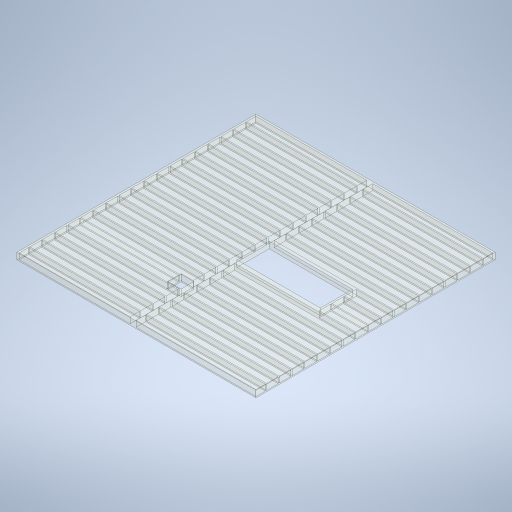
# Autodesk Inventor part: Existing_Basement_And_First_Floor_Transition
Saved by Autodesk Inventor 2024 (Build 280153000, 153)
## iProperties
Created: 2023-05-18
Part Number: Existing_Basement_And_First_Floor_Transition
Material: Wood (Southern Pine)
Document SubType Name: Modeling
Designer: Tom
Density: 7.85 g/cm^3
Appearance: Clear
Mass: 1.71886e+07 g
Surface Area: 1.80544e+06 cm^2
Volume: 2.18963e+06 cm^3
Author: Tom
Autodesk Inventor part; units mm, degrees
ref_plane "YZ Plane" through (0, 0, 0) normal (1, 0, 0) x (0, 1, 0)
ref_plane "XZ Plane" through (0, 0, 0) normal (0, 1, 0) x (-1, 0, 0)
ref_plane "XY Plane" through (0, 0, 0) normal (0, 0, 1) x (1, 0, 0)
sketch "Sketch1" plane through (0, 0, 0) normal (0, 1, 0) x (-1, 0, 0)
  line L0 (0, 0) -> (7620, 0)
  line L1 (7620, 0) -> (7620, -7620)
  line L2 (7620, -7620) -> (0, -7620)
  line L3 (0, -7620) -> (0, 0)
  line L4 (7581.9, -7581.9) -> (7581.9, -38.1)
  line L5 (7581.9, -38.1) -> (38.1, -38.1)
  line L6 (38.1, -38.1) -> (38.1, -7581.9)
  line L7 (38.1, -7581.9) -> (7581.9, -7581.9)
  line L8 (4051.3, -7581.9) -> (4051.3, -38.1)
  line L9 (3860.8, -38.1) -> (3860.8, -7581.9)
  line L10 (7581.9, -336.55) -> (38.1, -336.55)
  line L11 (38.1, -336.55) -> (38.1, -374.65)
  line L12 (38.1, -374.65) -> (7581.9, -374.65)
  line L13 (7581.9, -374.65) -> (7581.9, -336.55)
  line L14 (7581.9, -742.95) -> (38.1, -742.95)
  line L15 (38.1, -781.05) -> (7581.9, -781.05)
  line L16 (7581.9, -781.05) -> (7581.9, -742.95)
  line L17 (38.1, -742.95) -> (38.1, -781.05)
  line L18 (7581.9, -1149.35) -> (38.1, -1149.35)
  line L19 (38.1, -1187.45) -> (7581.9, -1187.45)
  line L20 (7581.9, -1187.45) -> (7581.9, -1149.35)
  line L21 (38.1, -1149.35) -> (38.1, -1187.45)
  line L22 (7581.9, -1555.75) -> (38.1, -1555.75)
  line L23 (38.1, -1593.85) -> (7581.9, -1593.85)
  line L24 (7581.9, -1593.85) -> (7581.9, -1555.75)
  line L25 (38.1, -1555.75) -> (38.1, -1593.85)
  line L26 (7581.9, -1962.15) -> (38.1, -1962.15)
  line L27 (38.1, -2000.25) -> (7581.9, -2000.25)
  line L28 (7581.9, -2000.25) -> (7581.9, -1962.15)
  line L29 (38.1, -1962.15) -> (38.1, -2000.25)
  line L30 (7581.9, -2368.55) -> (38.1, -2368.55)
  line L31 (38.1, -2406.65) -> (7581.9, -2406.65)
  line L32 (7581.9, -2406.65) -> (7581.9, -2368.55)
  line L33 (38.1, -2368.55) -> (38.1, -2406.65)
  line L34 (7581.9, -2774.95) -> (38.1, -2774.95)
  line L35 (38.1, -2813.05) -> (7581.9, -2813.05)
  line L36 (7581.9, -2813.05) -> (7581.9, -2774.95)
  line L37 (38.1, -2774.95) -> (38.1, -2813.05)
  line L38 (7581.9, -3181.35) -> (38.1, -3181.35)
  line L39 (38.1, -3219.45) -> (7581.9, -3219.45)
  line L40 (7581.9, -3219.45) -> (7581.9, -3181.35)
  line L41 (38.1, -3181.35) -> (38.1, -3219.45)
  line L42 (7581.9, -3587.75) -> (38.1, -3587.75)
  line L43 (38.1, -3625.85) -> (7581.9, -3625.85)
  line L44 (7581.9, -3625.85) -> (7581.9, -3587.75)
  line L45 (38.1, -3587.75) -> (38.1, -3625.85)
  line L46 (7581.9, -3994.15) -> (38.1, -3994.15)
  line L47 (38.1, -4032.25) -> (7581.9, -4032.25)
  line L48 (7581.9, -4032.25) -> (7581.9, -3994.15)
  line L49 (38.1, -3994.15) -> (38.1, -4032.25)
  line L50 (7581.9, -4400.55) -> (38.1, -4400.55)
  line L51 (38.1, -4438.65) -> (7581.9, -4438.65)
  line L52 (7581.9, -4438.65) -> (7581.9, -4400.55)
  line L53 (38.1, -4400.55) -> (38.1, -4438.65)
  line L54 (7581.9, -4806.95) -> (38.1, -4806.95)
  line L55 (38.1, -4845.05) -> (7581.9, -4845.05)
  line L56 (7581.9, -4845.05) -> (7581.9, -4806.95)
  line L57 (38.1, -4806.95) -> (38.1, -4845.05)
  line L58 (7581.9, -5213.35) -> (38.1, -5213.35)
  line L59 (38.1, -5251.45) -> (7581.9, -5251.45)
  line L60 (7581.9, -5251.45) -> (7581.9, -5213.35)
  line L61 (38.1, -5213.35) -> (38.1, -5251.45)
  line L62 (7581.9, -5619.75) -> (38.1, -5619.75)
  line L63 (38.1, -5657.85) -> (7581.9, -5657.85)
  line L64 (7581.9, -5657.85) -> (7581.9, -5619.75)
  line L65 (38.1, -5619.75) -> (38.1, -5657.85)
  line L66 (7581.9, -6026.15) -> (38.1, -6026.15)
  line L67 (38.1, -6064.25) -> (7581.9, -6064.25)
  line L68 (7581.9, -6064.25) -> (7581.9, -6026.15)
  line L69 (38.1, -6026.15) -> (38.1, -6064.25)
  line L70 (7581.9, -6432.55) -> (38.1, -6432.55)
  line L71 (38.1, -6470.65) -> (7581.9, -6470.65)
  line L72 (7581.9, -6470.65) -> (7581.9, -6432.55)
  line L73 (38.1, -6432.55) -> (38.1, -6470.65)
  line L74 (7581.9, -6838.95) -> (38.1, -6838.95)
  line L75 (38.1, -6877.05) -> (7581.9, -6877.05)
  line L76 (7581.9, -6877.05) -> (7581.9, -6838.95)
  line L77 (38.1, -6838.95) -> (38.1, -6877.05)
  line L78 (7581.9, -7245.35) -> (38.1, -7245.35)
  line L79 (38.1, -7283.45) -> (7581.9, -7283.45)
  line L80 (7581.9, -7283.45) -> (7581.9, -7245.35)
  line L81 (38.1, -7245.35) -> (38.1, -7283.45)
  point P0 (38.1, -7245.35)
  point P1 (38.1, -6838.95)
  point P2 (38.1, -6432.55)
  point P3 (38.1, -6026.15)
  point P4 (38.1, -5619.75)
  point P5 (38.1, -5213.35)
  point P6 (38.1, -4806.95)
  point P7 (38.1, -4400.55)
  point P8 (38.1, -3994.15)
  point P9 (38.1, -3587.75)
  point P10 (38.1, -3181.35)
  point P11 (38.1, -2774.95)
  point P12 (38.1, -2368.55)
  point P13 (38.1, -1962.15)
  point P14 (38.1, -1555.75)
  point P15 (38.1, -1149.35)
  point P16 (38.1, -742.95)
  point P17 (38.1, -336.55)
  point P18 (4051.3, -7283.45)
  point P19 (3860.8, -7283.45)
  point P20 (3860.8, -7245.35)
  point P21 (4051.3, -7245.35)
  point P22 (4051.3, -6877.05)
  point P23 (3860.8, -6877.05)
  point P24 (3860.8, -6838.95)
  point P25 (4051.3, -6838.95)
  point P26 (4051.3, -6470.65)
  point P27 (3860.8, -6470.65)
  point P28 (3860.8, -6432.55)
  point P29 (4051.3, -6432.55)
  point P30 (4051.3, -6064.25)
  point P31 (3860.8, -6064.25)
  point P32 (3860.8, -6026.15)
  point P33 (4051.3, -6026.15)
  point P34 (4051.3, -5657.85)
  point P35 (3860.8, -5657.85)
  point P36 (3860.8, -5619.75)
  point P37 (4051.3, -5619.75)
  point P38 (4051.3, -5251.45)
  point P39 (3860.8, -5251.45)
  point P40 (3860.8, -5213.35)
  point P41 (4051.3, -5213.35)
  point P42 (4051.3, -4845.05)
  point P43 (3860.8, -4845.05)
  point P44 (3860.8, -4806.95)
  point P45 (4051.3, -4806.95)
  point P46 (4051.3, -4438.65)
  point P47 (3860.8, -4438.65)
  point P48 (3860.8, -4400.55)
  point P49 (4051.3, -4400.55)
  point P50 (4051.3, -4032.25)
  point P51 (3860.8, -4032.25)
  point P52 (3860.8, -3994.15)
  point P53 (4051.3, -3994.15)
  point P54 (4051.3, -3625.85)
  point P55 (3860.8, -3625.85)
  point P56 (3860.8, -3587.75)
  point P57 (4051.3, -3587.75)
  point P58 (4051.3, -3219.45)
  point P59 (3860.8, -3219.45)
  point P60 (3860.8, -3181.35)
  point P61 (4051.3, -3181.35)
  point P62 (4051.3, -2813.05)
  point P63 (3860.8, -2813.05)
  point P64 (3860.8, -2774.95)
  point P65 (4051.3, -2774.95)
  point P66 (4051.3, -2406.65)
  point P67 (3860.8, -2406.65)
  point P68 (3860.8, -2368.55)
  point P69 (4051.3, -2368.55)
  point P70 (4051.3, -2000.25)
  point P71 (3860.8, -2000.25)
  point P72 (3860.8, -1962.15)
  point P73 (4051.3, -1962.15)
  point P74 (4051.3, -1593.85)
  point P75 (3860.8, -1593.85)
  point P76 (3860.8, -1555.75)
  point P77 (4051.3, -1555.75)
  point P78 (4051.3, -1187.45)
  point P79 (3860.8, -1187.45)
  point P80 (3860.8, -1149.35)
  point P81 (4051.3, -1149.35)
  point P82 (4051.3, -781.05)
  point P83 (3860.8, -781.05)
  point P84 (3860.8, -742.95)
  point P85 (4051.3, -742.95)
  point P86 (4051.3, -374.65)
  point P87 (3860.8, -374.65)
  point P88 (3860.8, -336.55)
  point P89 (4051.3, -336.55)
  dimension "d10" = 190.5
  dimension "d1" = 7620
  dimension "d3" = 7620
  dimension "d9" = 38.1
  dimension "d11" = 3568.7
  dimension "d12" = 38.1
  dimension "d13" = 336.55
  dimension "d16" = 406.4
  dimension "d21" = 336.55
  constraints: 156 end point, 68 vertical alignment, 39 parallel, 34 collinear, 5 horizontal, 4 point on line, 2 perpendicular, 17 other
  measures "d1" distance of L0.start L0.end
  measures "d3" distance of L2.end L0.start
  measures "d12" distance between parallel lines of L10 L12
  measures "d13" distance between parallel lines of L0 L10
  measures "d16" distance of L10.start L14.start
  measures "d21" distance between parallel lines of L2 L79
extrude "Extrusion1" add sketch "Sketch1" along normal blind 190.5 contours L0 L1 L2 L3 | L79 L8 L78 L4 | L7 L9 L79 L8 | L79 L9 L78 L8 | L75 L8 L74 L4 | L78 L9 L75 L8 | L79 L6 L78 L9 | L75 L9 L74 L8 | L71 L8 L70 L4 | L74 L9 L71 L8 | L75 L6 L74 L9 | L71 L9 L70 L8 | L67 L8 L66 L4 | L70 L9 L67 L8 | L71 L6 L70 L9 | L67 L9 L66 L8 | L63 L8 L62 L4 | L66 L9 L63 L8 | L67 L6 L66 L9 | L63 L9 L62 L8 | L59 L8 L58 L4 | L62 L9 L59 L8 | L63 L6 L62 L9 | L59 L9 L58 L8 | L55 L8 L54 L4 | L58 L9 L55 L8 | L59 L6 L58 L9 | L55 L9 L54 L8 | L51 L8 L50 L4 | L54 L9 L51 L8 | L55 L6 L54 L9 | L51 L9 L50 L8 | L47 L8 L46 L4 | L50 L9 L47 L8 | L51 L6 L50 L9 | L47 L9 L46 L8 | L43 L8 L42 L4 | L46 L9 L43 L8 | L47 L6 L46 L9 | L43 L9 L42 L8 | L39 L8 L38 L4 | L42 L9 L39 L8 | L43 L6 L42 L9 | L39 L9 L38 L8 | L35 L8 L34 L4 | L38 L9 L35 L8 | L39 L6 L38 L9 | L35 L9 L34 L8 | L31 L8 L30 L4 | L34 L9 L31 L8 | L35 L6 L34 L9 | L31 L9 L30 L8 | L27 L8 L26 L4 | L30 L9 L27 L8 | L31 L6 L30 L9 | L27 L9 L26 L8 | L23 L8 L22 L4 | L26 L9 L23 L8 | L27 L6 L26 L9 | L23 L9 L22 L8 | L19 L8 L18 L4 | L22 L9 L19 L8 | L23 L6 L22 L9 | L19 L9 L18 L8 | L15 L8 L14 L4 | L18 L9 L15 L8 | L19 L6 L18 L9 | L15 L9 L14 L8 | L12 L8 L10 L4 | L14 L9 L12 L8 | L15 L6 L14 L9 | L12 L9 L10 L8 | L10 L9 L5 L8 | L12 L6 L10 L9
sketch "Sketch2" plane through (0, 190.5, 0) normal (0, 1, 0) x (1, 0, 0)
  line L0 (-7620, 7620) -> (-7620, 0) projected
  line L1 (-7620, 7620) -> (0, 7620)
  line L2 (0, 7620) -> (0, 0)
  line L3 (0, 0) -> (-7620, 0)
  line L4 (-7620, 0) -> (-7620, 7620)
  constraints: 8 end point, 2 parallel, 1 horizontal, 1 perpendicular
extrude "Extrusion2" add sketch "Sketch2" along normal blind 19.05
sketch "Sketch3" plane through (0, 209.55, 0) normal (0, 1, 0) x (1, 0, 0)
  line L0 (-3987.8, 2006.6) -> (-4394.2, 2006.6)
  line L1 (-4394.2, 2006.6) -> (-4394.2, 1600.2)
  line L2 (-4394.2, 1600.2) -> (-3987.8, 1600.2)
  line L3 (-3987.8, 1600.2) -> (-3987.8, 2006.6)
  line L4 (-7620, 0) -> (0, 0) projected
  point P0 (-7581.9, 742.95)
  dimension "d25" = 406.4
  dimension "d26" = 406.4
  dimension "d27" = 3187.7
  dimension "d28" = 1600.2
  constraints: 8 end point, 2 parallel, 1 horizontal, 1 perpendicular
  measures "d25" distance between parallel lines of L2 L0
  measures "d26" distance between parallel lines of L3 L1
  measures "d27" distance from line of point (-7581.9, 742.95) L1
  measures "d28" distance between parallel lines of L4 L2
extrude "Extrusion3" cut sketch "Sketch3" against normal blind 19.05
sketch "Sketch4" plane through (0, 209.55, 0) normal (0, 1, 0) x (1, 0, 0)
  line L0 (-1244.6, 3295.65) -> (-3905.25, 3295.65)
  line L1 (-3905.25, 3295.65) -> (-3905.25, 4324.35)
  line L2 (-3905.25, 4324.35) -> (-1244.6, 4324.35)
  line L3 (-1244.6, 4324.35) -> (-1244.6, 3295.65)
  line L4 (0, 0) -> (0, 7620) projected
  line L5 (-7620, 0) -> (0, 0) projected
  point P0 (-1244.6, 3810)
  dimension "d32" = 2660.65
  dimension "d33" = 3295.65
  dimension "d34" = 1028.7
  dimension "d45" = 3905.25
  constraints: 8 end point, 2 parallel, 1 horizontal, 1 midpoint, 1 perpendicular
  measures "d32" distance of L0.start L0.end
  measures "d33" distance between parallel lines of L5 L0
  measures "d34" distance of L2.end L0.start
  measures "d45" distance between parallel lines of L4 L1
extrude "Extrusion4" cut sketch "Sketch4" against normal through all
sketch "Sketch8" plane through (0, 0, 0) normal (0, -1, 0) x (1, 0, 0)
  line L0 (-1244.6, -3587.75) -> (-38.1, -3587.75) projected
  line L1 (-1206.5, -3587.75) -> (-1244.6, -3587.75)
  line L2 (-1244.6, -3587.75) -> (-1244.6, -3219.45)
  line L3 (-1206.5, -3219.45) -> (-1206.5, -3587.75)
  line L4 (-38.1, -3625.85) -> (-1244.6, -3625.85) projected
  line L5 (-1244.6, -3625.85) -> (-1244.6, -3994.15) projected
  line L6 (-1206.5, -3625.85) -> (-1244.6, -3625.85)
  line L7 (-1244.6, -3625.85) -> (-1244.6, -3994.15)
  line L8 (-1244.6, -3994.15) -> (-1206.5, -3994.15)
  line L9 (-1206.5, -3994.15) -> (-1206.5, -3625.85)
  line L10 (-1206.5, -4032.25) -> (-1244.6, -4032.25)
  line L11 (-1244.6, -4032.25) -> (-1244.6, -4400.55)
  line L12 (-1244.6, -4400.55) -> (-1206.5, -4400.55)
  line L13 (-1206.5, -4400.55) -> (-1206.5, -4032.25)
  line L14 (-1244.6, -3295.65) -> (-1244.6, -3587.75) projected
  line L15 (-38.1, -3219.45) -> (-3860.8, -3219.45) projected
  line L16 (-1244.6, -3219.45) -> (-1206.5, -3219.45)
  line L17 (-3860.8, -4400.55) -> (-38.1, -4400.55) projected
  line L18 (-38.1, -4032.25) -> (-1244.6, -4032.25) projected
  line L19 (-1244.6, -3295.65) -> (-3860.8, -3295.65)
  line L20 (-3860.8, -3295.65) -> (-3860.8, -3219.45)
  line L21 (-3860.8, -3219.45) -> (-1244.6, -3219.45)
  line L22 (-1244.6, -3219.45) -> (-1244.6, -3295.65)
  line L23 (-1244.6, -4324.35) -> (-3860.8, -4324.35) projected
  line L24 (-1244.6, -4400.55) -> (-3860.8, -4400.55)
  line L25 (-3860.8, -4400.55) -> (-3860.8, -4324.35)
  line L26 (-3860.8, -4324.35) -> (-1244.6, -4324.35)
  line L27 (-1244.6, -4324.35) -> (-1244.6, -4400.55)
  point P0 (0, 0)
  dimension "d46" = 38.1
  constraints: 40 end point, 9 parallel, 6 point on line, 5 horizontal, 5 perpendicular, 4 collinear
  measures "d46" distance between parallel lines of L7 L9
extrude "Extrusion8" add sketch "Sketch8" against normal blind 190.5
sketch "Sketch9" plane through (0, 209.55, 0) normal (0, 1, 0) x (1, 0, 0)
  line L0 (-4394.2, 2006.6) -> (-3987.8, 2006.6) projected
  line L1 (-3987.8, 1600.2) -> (-4394.2, 1600.2) projected
  line L2 (-4394.2, 2006.6) -> (-3987.8, 2006.6)
  line L3 (-3987.8, 2006.6) -> (-3987.8, 1600.2)
  line L4 (-3987.8, 1600.2) -> (-4394.2, 1600.2)
  line L5 (-4394.2, 1600.2) -> (-4394.2, 2006.6)
  point P0 (0, 0)
  constraints: 8 end point, 2 parallel, 1 horizontal, 1 perpendicular
extrude "Extrusion9" cut sketch "Sketch9" against normal up to surface (209.55 mm away)
sketch "Sketch10" plane through (0, 0, 0) normal (0, -1, 0) x (1, 0, 0)
  line L0 (-4394.2, -1962.15) -> (-4394.2, -1600.2) projected
  line L1 (-7581.9, -1962.15) -> (-4394.2, -1962.15) projected
  line L2 (-4394.2, -1600.2) -> (-4432.3, -1600.2)
  line L3 (-4432.3, -1600.2) -> (-4432.3, -1962.15)
  line L4 (-4432.3, -1962.15) -> (-4394.2, -1962.15)
  line L5 (-4394.2, -1962.15) -> (-4394.2, -1600.2)
  line L6 (-4051.3, -2006.6) -> (-4394.2, -2006.6) projected
  line L7 (-4051.3, -2006.6) -> (-4432.3, -2006.6)
  line L8 (-4432.3, -2006.6) -> (-4432.3, -2044.7)
  line L9 (-4432.3, -2044.7) -> (-4051.3, -2044.7)
  line L10 (-4051.3, -2044.7) -> (-4051.3, -2006.6)
  line L11 (-4394.2, -2000.25) -> (-7581.9, -2000.25) projected
  line L12 (-4432.3, -2006.6) -> (-4394.2, -2006.6)
  line L13 (-4394.2, -2006.6) -> (-4394.2, -2000.25)
  line L14 (-4394.2, -2000.25) -> (-4432.3, -2000.25)
  line L15 (-4432.3, -2000.25) -> (-4432.3, -2006.6)
  point P0 (0, 0)
  dimension "d51" = 38.1
  constraints: 24 end point, 6 parallel, 4 perpendicular, 3 horizontal, 2 point on line
  measures "d51" distance between parallel lines of L3 L0
extrude "Extrusion10" add sketch "Sketch10" against normal blind 190.5
body "Solid1"
